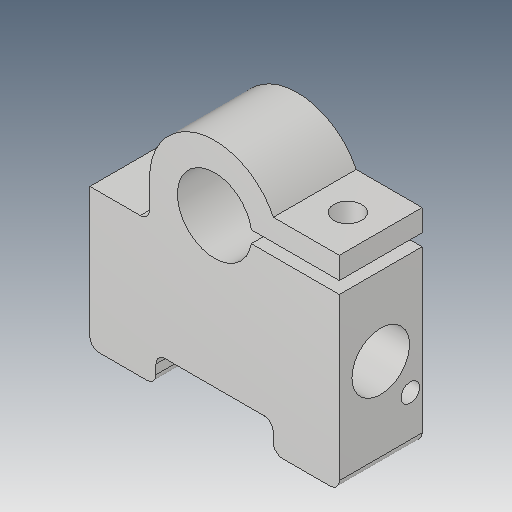
# Autodesk Inventor part: hotend
Saved by Autodesk Inventor 2019 (Build 230136000, 136)
## iProperties
Created: 2018-11-13
Part Number: hotend
Material: Aluminum
Document SubType Name: Modeling
Designer: LillaHunden
Density: 2.7 g/cm^3
Appearance: Satin
Mass: 8.88803 g
Surface Area: 30.0331 cm^2
Volume: 3.29186 cm^3
Author: LillaHunden
Autodesk Inventor part; units mm, degrees
ref_plane "YZ Plane" through (0, 0, 0) normal (1, 0, 0) x (0, 1, 0)
ref_plane "XZ Plane" through (0, 0, 0) normal (0, 1, 0) x (-1, 0, 0)
ref_plane "XY Plane" through (0, 0, 0) normal (0, 0, 1) x (1, 0, 0)
sketch "Sketch1" plane through (0, 0, 0) normal (0, 0, 1) x (1, 0, 0)
  line L0 (-13.425, -7.5) -> (13.425, -7.5)
  line L1 (13.425, -7.5) -> (13.425, 7.5)
  line L2 (13.425, 7.5) -> (-13.425, 7.5)
  line L3 (-13.425, 7.5) -> (-13.425, -7.5)
  line L4 (-13.425, -7.5) -> (13.425, 7.5) construction
  line L5 (13.425, -7.5) -> (-13.425, 7.5) construction
  point P0 (0, 0)
  dimension "d0" = 26.85
  dimension "d1" = 15
  constraints: 12 end point, 2 midpoint, 2 parallel, 1 horizontal, 1 perpendicular
  measures "d0" distance of L2.end L1.end
  measures "d1" distance of L1.end L0.end
extrude "Extrusion1" add sketch "Sketch1" along normal blind 8.91
sketch "Sketch2" plane through (0, 0, 8.91) normal (0, 0, 1) x (1, 0, 0)
  line L0 (-13.425, -7.5) -> (13.425, -7.5) projected
  line L1 (-6.315, -7.5) -> (6.315, -7.5)
  line L2 (6.315, -7.5) -> (6.315, -4.5)
  line L3 (6.315, -4.5) -> (-6.315, -4.5)
  line L4 (-6.315, -4.5) -> (-6.315, -7.5)
  line L5 (-13.425, 7.5) -> (-13.425, -7.5) projected
  line L6 (13.425, -7.5) -> (13.425, 7.5) projected
  point P0 (0, 0)
  dimension "d4" = 7.11
  dimension "d5" = 7.11
  dimension "d6" = 3
  constraints: 8 end point, 2 parallel, 1 horizontal, 1 perpendicular, 1 point on line
  measures "d4" distance between parallel lines of L5 L4
  measures "d5" distance between parallel lines of L6 L2
  measures "d6" distance between parallel lines of L0 L3
extrude "Extrusion2" cut sketch "Sketch2" against normal through all
fillet "Fillet1" radius 1 6 edges at (-6.315, -4.5, 4.455) (6.315, -4.5, 4.455) (6.315, -7.5, 4.455) (-6.315, -7.5, 4.455) (-13.425, -7.5, 4.455) (13.425, -7.5, 4.455)
hole "Hole1" at (-9.87, -7.5, 4.455) direction (0, 1, 0) diameter 2.459 depth 5.05 tip angle 118 thread size "M3x0.5" class "6H" standard "ISO Metric profile"
hole "Hole2" at (9.87, -7.5, 4.455) direction (0, 1, 0) diameter 2.459 depth 5.05 tip angle 118 thread size "M3x0.5" class "6H" standard "ISO Metric profile"
sketch "Sketch3" plane through (-13.425, 7.5, 0) normal (-1, 0, 0) x (0, 0, 1)
  circle A0 centre (4.455, -5.1) radius 3.1
  line L0 (6.8136, -2) -> (2.7173, -2)
  line L1 (0, -15) -> (8.91, -15) projected
  point P0 (0, -7.5)
  point P1 (4.455, -15)
  dimension "d28" = 6.2
  dimension "d29" = 13
  constraints: 2 end point, 1 centre point, 1 horizontal, 1 midpoint, 1 tangent, 1 vertical alignment
  measures "d28" diameter of A0
  measures "d29" distance between parallel lines of L1 L0
extrude "Extrusion3" cut sketch "Sketch3" against normal through all
sketch "Sketch4" plane through (-13.425, 7.5, 0) normal (-1, 0, 0) x (0, 0, 1)
  circle A0 centre (1.2775, -9.6) radius 1
  line L0 (0, -15) -> (8.91, -15) projected
  point P0 (0, -7.5)
  dimension "d32" = 2
  dimension "d33" = 5.4
  constraints: 1 centre point
  measures "d32" diameter of A0
  measures "d33" distance from line of L0 A0.centre
extrude "Extrusion4" cut sketch "Sketch4" against normal through all
sketch "Sketch5" plane through (0, 0, 8.91) normal (0, 0, 1) x (1, 0, 0)
  line L0 (13.425, 7.5) -> (-13.425, 7.5) projected
  line L1 (-5.315, -4.5) -> (5.315, -4.5) projected
  line L2 (-7, 11.5) -> (-7, 7.5)
  line L3 (13.425, -6.5) -> (13.425, 7.5) projected
  line L4 (13.425, 14.5) -> (6.3246, 14.5)
  line L5 (7, 11.5) -> (13.425, 11.5) construction
  line L6 (7.315, -7.5) -> (12.425, -7.5) projected
  line L7 (13.425, 7.5) -> (13.425, 10.87)
  line L8 (13.425, 12.13) -> (13.425, 14.5)
  arc A0 (6.3246, 14.5) -> (-7, 11.5) centre (0, 11.5) ccw
  line L9 (-7, 7.5) -> (13.425, 7.5)
  line L10 (13.425, 12.13) -> (13.425, 10.87)
  point P0 (0, 0)
  dimension "d40" = 22
  constraints: 14 end point, 3 vertical, 2 point on circle, 1 centre point, 1 collinear, 1 horizontal alignment, 1 point on line, 1 tangent
  measures "d40" distance between parallel lines of L6 L4
extrude "Extrusion5" add sketch "Sketch5" against normal up to surface (8.91 mm away)
sketch "Sketch6" plane through (0, 0, 8.91) normal (0, 0, 1) x (1, 0, 0)
  arc A0 (6.3246, 14.5) -> (-7, 11.5) centre (0, 11.5) ccw projected
  circle A1 centre (0, 11.5) radius 4
  point P0 (0, 0)
  dimension "d43" = 8
  constraints: 1 centre point, 1 coincident
  measures "d43" diameter of A1
extrude "Extrusion6" cut sketch "Sketch6" against normal through all
sketch "Sketch7" plane through (0, 0, 8.91) normal (0, 0, 1) x (1, 0, 0)
  line L0 (2.5936, 12.15) -> (18.1554, 12.15)
  line L1 (18.1554, 12.15) -> (18.1554, 10.85)
  line L2 (18.1554, 10.85) -> (2.5936, 10.85)
  line L3 (2.5936, 10.85) -> (2.5936, 12.15)
  circle A0 centre (0, 11.5) radius 4 construction
  point P0 (0, 0)
  point P1 (2.5936, 11.5)
  dimension "d46" = 1.3
  constraints: 8 end point, 2 parallel, 1 horizontal, 1 horizontal alignment, 1 midpoint, 1 perpendicular
  measures "d46" distance of L2.end L0.start
extrude "Extrusion7" cut sketch "Sketch7" against normal through all
fillet "Fillet2" radius 1 1 edges at (-7, 7.5, 4.455)
hole "Hole3" at (9.8748, 14.5, 4.455) direction (0, -1, 0) diameter 3 depth 5.8 tip angle 118
thread "Thread1" size "M3x0.5" class "6H" standard "ANSI Metric M Profile" full length
hole "Hole4" at (0, -4.5, 4.455) direction (0, 1, 0) diameter 2.013 depth 6.35 tip angle 118 thread size "M2.5x0.45" class "6H" standard "ISO Metric profile"
equation "\"d5\" = d4"
body "Solid1"
